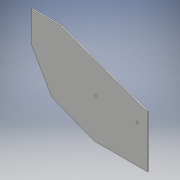
# Autodesk Inventor part: endplate
Saved by Autodesk Inventor 2018.3 (Build 223284000, 284)
## iProperties
Created: 2018-06-13
Part Number: endplate
Material: 一般
Document SubType Name: Modeling
Designer: ku_sk
Density: 1 g/cm^3
Appearance: 既定
Author: ku_sk
Autodesk Inventor part; units mm, degrees
ref_plane "YZ Plane" through (0, 0, 0) normal (1, 0, 0) x (0, 1, 0)
ref_plane "XZ Plane" through (0, 0, 0) normal (0, 1, 0) x (-1, 0, 0)
ref_plane "XY Plane" through (0, 0, 0) normal (0, 0, 1) x (1, 0, 0)
sketch "スケッチ3" plane through (0, 0, 0) normal (0, 1, 0) x (-1, 0, 0)
  line L0 (254.1154, -190) -> (474.1154, -103.3975) projected
  line L1 (254.1154, -190) -> (-20, -190) projected
  line L2 (-20, -190) -> (-20, 80) projected
  line L3 (-20, 80) -> (430, 240) projected
  line L4 (430, 240) -> (580, 240) projected
  line L5 (580, 240) -> (580, 80) projected
  line L6 (580, 80) -> (474.1154, -103.3975) projected
  circle A0 centre (420, 145) radius 2.5 projected
  circle A1 centre (320, 75) radius 2.5 projected
  circle A2 centre (0, 0) radius 2.5 projected
  circle A3 centre (247.4696, 17.1833) radius 6 projected
  circle A4 centre (32.803, 5.2135) radius 6 projected
  point P0 (0, 0)
extrude "押し出し1" add sketch "スケッチ3" along normal mid plane 6 contours L1 L2 L3 L4 L5 L6 L0 | A0 | A1 | A2
sketch "スケッチ4" plane through (0, -3, 0) normal (0, -1, 0) x (1, 0, 0)
  circle A0 centre (-247.4696, 17.1833) radius 6 projected
  circle A1 centre (-32.803, 5.2135) radius 6 projected
  circle A2 centre (-247.4696, 17.1833) radius 4.5
  circle A3 centre (-32.803, 5.2135) radius 4.5
  point P0 (0, 0)
  dimension "d4" = 9
  dimension "d5" = 9
  constraints: 2 centre point, 2 coincident
  measures "d4" diameter of A2
  measures "d5" diameter of A3
extrude "押し出し2" add sketch "スケッチ4" against normal blind 6
